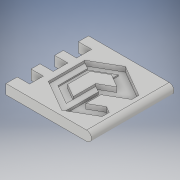
# Autodesk Inventor part: schablone
Saved by Autodesk Inventor 2019 (Build 230136000, 136)
## iProperties
Created: 2019-08-14
Part Number: schablone
Material: Generic
Document SubType Name: Modeling
Designer: Yashar
Density: 1 g/cm^3
Appearance: Default
Author: Yashar
Autodesk Inventor part; units mm, degrees
note: some values were not read from the file. Chosen so that the rebuilt part matches the saved one: direction of "Emboss1".
ref_plane "YZ Plane" through (0, 0, 0) normal (1, 0, 0) x (0, 1, 0)
ref_plane "XZ Plane" through (0, 0, 0) normal (0, 1, 0) x (-1, 0, 0)
ref_plane "XY Plane" through (0, 0, 0) normal (0, 0, 1) x (1, 0, 0)
sketch "Sketch1" plane through (0, 0, 0) normal (0, 1, 0) x (-1, 0, 0)
  line L0 (-17.5, 16.9) -> (17.5, 16.9)
  line L1 (17.5, 16.9) -> (17.5, -16.9)
  line L2 (17.5, -16.9) -> (-17.5, -16.9)
  line L3 (-17.5, -16.9) -> (-17.5, 16.9)
  line L4 (-17.5, 16.9) -> (17.5, -16.9) construction
  line L5 (17.5, 16.9) -> (-17.5, -16.9) construction
  point P0 (0, 0)
  constraints: 12 end point, 2 midpoint, 2 parallel, 1 horizontal, 1 perpendicular
sketch "Sketch2" plane through (0, 0, 0) normal (0, 1, 0) x (-1, 0, 0)
  line L0 (980.2308, 0) -> (977.7308, 0)
  line L1 (17.4632, -0.049) -> (15.105, -0.049)
  line L2 (12.1095, 2.9465) -> (18.1005, 2.9465)
  line L3 (18.1005, 2.9465) -> (18.1005, -3.0446)
  line L4 (18.1005, -3.0446) -> (12.1095, -3.0446)
  line L5 (12.1095, -3.0446) -> (12.1095, 2.9465)
  line L6 (12.1095, 2.9465) -> (18.1005, -3.0446) construction
  line L7 (18.1005, 2.9465) -> (12.1095, -3.0446) construction
  line L8 (12.4632, 12.2678) -> (18.1005, 12.2678)
  line L9 (18.1005, 12.2678) -> (18.1005, 6.638)
  line L10 (18.1005, 6.638) -> (12.4632, 6.638)
  line L11 (12.4632, 6.638) -> (12.4632, 12.2678)
  line L12 (12.4632, 12.2678) -> (18.1005, 6.638) construction
  line L13 (12.0658, -6.5864) -> (18.1005, -6.5864)
  line L14 (18.1005, -6.5864) -> (18.1005, -12.7382)
  line L15 (18.1005, -12.7382) -> (12.0658, -12.7382)
  line L16 (12.0658, -12.7382) -> (12.0658, -6.5864)
  line L17 (12.0658, -6.5864) -> (18.1005, -12.7382) construction
  line L18 (18.1005, -6.5864) -> (12.0658, -12.7382) construction
  point P0 (0, 0)
  dimension "d2" = 2.5
  constraints: 38 end point, 6 parallel, 5 horizontal, 3 perpendicular, 2 midpoint
  measures "d2" distance of L0.start L0.end
extrude "Extrusion1" add sketch "Sketch1" along normal blind 4
extrude "Extrusion2" cut sketch "Sketch2" along normal blind 4
fillet "Fillet3" radius 2 1 edges at (17.5, 4, 0)
fillet "Fillet4" radius 2 1 edges at (17.5, 0, 0)
sketch "Sketch3" plane through (0, 4, 0) normal (0, 1, 0) x (1, 0, 0)
  line L0 (-17.5, 3.0446) -> (-12.1095, 3.0446) construction
  line L1 (-12.1095, 3.0446) -> (-12.1095, -2.9465) construction
  line L2 (-12.1095, -2.9465) -> (-17.5, -2.9465) construction
  line L3 (-17.5, -2.9465) -> (-17.5, -6.638) construction
  line L4 (-17.5, -6.638) -> (-12.4632, -6.638) construction
  line L5 (-12.4632, -6.638) -> (-12.4632, -12.2678) construction
  line L6 (-12.4632, -12.2678) -> (-17.5, -12.2678) construction
  line L7 (-17.5, -12.2678) -> (-17.5, -16.9) construction
  line L8 (-17.5, -16.9) -> (15.5, -16.9) construction
  line L9 (15.5, 16.9) -> (-17.5, 16.9) construction
  line L10 (-17.5, 16.9) -> (-17.5, 12.7382) construction
  line L11 (-17.5, 12.7382) -> (-12.0658, 12.7382) construction
  line L12 (-12.0658, 12.7382) -> (-12.0658, 6.5864) construction
  line L13 (-12.0658, 6.5864) -> (-17.5, 6.5864) construction
  line L14 (-17.5, 6.5864) -> (-17.5, 3.0446) construction
  line L15 (-12.1095, 0.049) -> (15.5, 0) construction
  line L16 (-17.5, 16.9) -> (17.5, 16.9) construction
  line L17 (17.5, -16.9) -> (-17.5, -16.9) construction
  line L18 (-9.5803, 7.5215) -> (-9.5803, -7.4785)
  line L19 (-9.5803, -7.4785) -> (3.41, -14.9785)
  line L20 (-9.5803, 7.5215) -> (-7.0803, 6.0781)
  line L21 (-7.0803, 6.0781) -> (-7.0803, -6.0352)
  line L22 (-7.0803, -6.0352) -> (0.91, -10.6484)
  line L23 (0.91, -10.6484) -> (0.91, 1.4648)
  line L24 (0.91, 1.4648) -> (3.41, 0.0215)
  line L25 (3.41, 0.0215) -> (3.41, -14.9785)
  line L26 (15.5, 16.9) -> (15.5, -16.9) projected
  line L27 (3.41, 16.9) -> (3.41, -16.9) construction
  line L28 (-17.5, -16.9) -> (15.5, -16.9) construction
  line L29 (15.5, 16.9) -> (15.5, 16.9) construction
  line L30 (15.5, 16.9) -> (15.5, -16.9) construction
  line L31 (15.5, -16.9) -> (15.5, -16.9) construction
  line L32 (15.5, -16.9) -> (15.5, 16.9) construction
  dimension "d23" = 2.5
  dimension "d24" = 2.5
  dimension "d25" = 2.5
  dimension "d26" = 15
  dimension "d28" = 15
  constraints: 20 end point, 4 parallel, 3 collinear, 3 point on line, 2 midpoint, 1 perpendicular, 1 vertical
  measures "d23" distance between parallel lines of L21 L18
  measures "d24" distance between parallel lines of L25 L23
  measures "d25" distance between parallel lines of L19 L22
  measures "d26" distance of L18.start L18.end
  measures "d28" distance of L18.end L19.end
emboss "Emboss1" sketch "Sketch3" operation cut depth 1 direction (0, -1, 0)
sketch "Sketch4" plane through (0, 4, 0) normal (0, 1, 0) x (1, 0, 0)
  line L0 (-9.5803, 7.5215) -> (-7.0803, 6.0781) construction
  line L1 (-7.0803, 6.0781) -> (-7.0803, -6.0352) construction
  line L2 (-7.0803, -6.0352) -> (0.91, -10.6484) construction
  line L3 (0.91, -10.6484) -> (0.91, 1.4648) construction
  line L4 (0.91, 1.4648) -> (3.41, 0.0215) construction
  line L5 (3.41, 0.0215) -> (3.41, -14.9785) construction
  line L6 (3.41, -14.9785) -> (-9.5803, -7.4785) construction
  line L7 (-9.5803, -7.4785) -> (-9.5803, 7.5215) construction
  line L8 (15.5, 16.9) -> (15.5, -16.9) construction
  line L9 (15.5, 16.9) -> (-17.5, 16.9) construction
  line L10 (-17.5, 16.9) -> (-17.5, 12.7382) construction
  line L11 (-17.5, 12.7382) -> (-12.0658, 12.7382) construction
  line L12 (-12.0658, 12.7382) -> (-12.0658, 6.5864) construction
  line L13 (-12.0658, 6.5864) -> (-17.5, 6.5864) construction
  line L14 (-17.5, 6.5864) -> (-17.5, 3.0446) construction
  line L15 (-17.5, 3.0446) -> (-12.1095, 3.0446) construction
  line L16 (-12.1095, 3.0446) -> (-12.1095, -2.9465) construction
  line L17 (-12.1095, -2.9465) -> (-17.5, -2.9465) construction
  line L18 (-17.5, -2.9465) -> (-17.5, -6.638) construction
  line L19 (-17.5, -6.638) -> (-12.4632, -6.638) construction
  line L20 (-12.4632, -6.638) -> (-12.4632, -12.2678) construction
  line L21 (-12.4632, -12.2678) -> (-17.5, -12.2678) construction
  line L22 (-17.5, -12.2678) -> (-17.5, -16.9) construction
  line L23 (-17.5, -16.9) -> (15.5, -16.9) construction
  line L24 (-12.1095, 0.049) -> (15.5, 0) construction
  line L25 (15.5, -16.9) -> (15.5, 16.9) construction
  line L26 (0.91, 16.9) -> (0.91, -16.9) construction
  line L27 (15.5, -16.9) -> (-17.5, -16.9) construction
  line L28 (0.91, -10.6484) -> (0.91, 1.4648) construction
  line L29 (-7.0803, 6.0781) -> (-7.0803, -6.0352) projected
  line L30 (-7.0803, -6.0352) -> (0.91, -10.6484) projected
  line L31 (-7.0803, 6.0781) -> (-7.0803, -6.0352)
  line L32 (-7.0803, -6.0352) -> (0.91, -10.6484)
  line L33 (0.91, -10.6484) -> (0.91, -7.7617)
  line L34 (0.91, -10.6484) -> (0.91, 1.4648) projected
  line L35 (0.91, -7.7617) -> (-4.5803, -4.5918)
  line L36 (-4.5803, -4.5918) -> (-4.5803, 4.6347)
  line L37 (-4.5803, 4.6347) -> (0.91, 7.8046)
  line L38 (-7.0803, 6.0781) -> (0.91, 10.6913)
  line L39 (0.91, 10.6913) -> (0.91, 7.8046)
  point P0 (0, 0)
  dimension "d29" = 120
  dimension "d30" = 2.5
  dimension "d31" = 2.5
  dimension "d32" = 2.5
  constraints: 20 end point, 5 point on line, 4 collinear, 4 parallel, 2 midpoint
  measures "d29" angle of L38 L0
  measures "d30" distance between parallel lines of L1 L36
  measures "d31" distance between parallel lines of L38 L37
  measures "d32" distance between parallel lines of L2 L35
emboss "Emboss2" sketch "Sketch4" operation cut depth 1.5 direction (0, -1, 0)
sketch "Sketch5" plane through (0, 4, 0) normal (0, 1, 0) x (1, 0, 0)
  line L0 (-4.5803, -4.5918) -> (0.91, -7.7617) construction
  line L1 (0.91, -7.7617) -> (0.91, 1.4648) construction
  line L2 (0.91, 1.4648) -> (3.41, 0.0215) construction
  line L3 (3.41, 0.0215) -> (3.41, -14.9785) construction
  line L4 (3.41, -14.9785) -> (-9.5803, -7.4785) construction
  line L5 (-9.5803, -7.4785) -> (-9.5803, 7.5215) construction
  line L6 (-9.5803, 7.5215) -> (-7.0803, 6.0781) construction
  line L7 (-7.0803, 6.0781) -> (0.91, 10.6913) construction
  line L8 (0.91, 10.6913) -> (0.91, 7.8046) construction
  line L9 (0.91, 7.8046) -> (-4.5803, 4.6347) construction
  line L10 (-4.5803, 4.6347) -> (-4.5803, -4.5918) construction
  line L11 (15.5, 16.9) -> (15.5, -16.9) construction
  line L12 (15.5, 16.9) -> (-17.5, 16.9) construction
  line L13 (-17.5, 16.9) -> (-17.5, 12.7382) construction
  line L14 (-17.5, 12.7382) -> (-12.0658, 12.7382) construction
  line L15 (-12.0658, 12.7382) -> (-12.0658, 6.5864) construction
  line L16 (-12.0658, 6.5864) -> (-17.5, 6.5864) construction
  line L17 (-17.5, 6.5864) -> (-17.5, 3.0446) construction
  line L18 (-17.5, 3.0446) -> (-12.1095, 3.0446) construction
  line L19 (-12.1095, 3.0446) -> (-12.1095, -2.9465) construction
  line L20 (-12.1095, -2.9465) -> (-17.5, -2.9465) construction
  line L21 (-17.5, -2.9465) -> (-17.5, -6.638) construction
  line L22 (-17.5, -6.638) -> (-12.4632, -6.638) construction
  line L23 (-12.4632, -6.638) -> (-12.4632, -12.2678) construction
  line L24 (-12.4632, -12.2678) -> (-17.5, -12.2678) construction
  line L25 (-17.5, -12.2678) -> (-17.5, -16.9) construction
  line L26 (-17.5, -16.9) -> (15.5, -16.9) construction
  line L27 (-7.0803, 6.0781) -> (0.91, 10.6913) projected
  line L28 (-9.5803, 7.5215) -> (-7.0803, 6.0781)
  line L29 (-7.0803, 6.0781) -> (0.91, 10.6913)
  line L30 (0.91, 10.6913) -> (0.91, 7.8046)
  line L31 (0.91, 10.6913) -> (0.91, 7.8046) projected
  line L32 (0.91, 16.9) -> (0.91, -16.9) construction
  line L33 (0.91, -7.7617) -> (0.91, 1.4648) construction
  line L34 (-9.5803, 7.5215) -> (0.91, 13.5781)
  line L35 (0.91, 13.5781) -> (13.9004, 6.0781)
  line L36 (13.9004, 6.0781) -> (13.9004, 3.1913)
  line L37 (13.9004, 3.1913) -> (5.91, -1.4219)
  line L38 (5.91, -1.4219) -> (5.91, -7.6363)
  line L39 (5.91, -7.6363) -> (11.2919, -4.5291)
  line L40 (13.9004, -6.0352) -> (13.9004, -8.9219)
  line L41 (3.41, -14.9785) -> (-9.5803, -7.4785) projected
  line L42 (13.9004, -8.9219) -> (3.41, -14.9785)
  line L43 (0.91, 1.4648) -> (3.41, 0.0215) projected
  line L44 (3.41, -14.9785) -> (3.41, 0.0215)
  line L45 (3.41, 0.0215) -> (0.91, 1.4648)
  line L46 (0.91, 7.8046) -> (-4.5803, 4.6347) projected
  line L47 (0.91, 7.8046) -> (0.91, 10.6913)
  line L48 (3.41, 0.0215) -> (3.41, -14.9785) projected
  line L49 (0.91, 1.4648) -> (6.4004, 4.6347)
  line L50 (6.4004, 4.6347) -> (0.91, 7.8046)
  line L51 (13.9004, -6.0352) -> (11.2919, -4.5291)
  line L52 (-7.1521, -6.1594) -> (3.41, -12.0918) construction
  line L53 (-4.5803, -4.5918) -> (0.91, -7.7617) construction
  line L54 (-4.5803, -4.5918) -> (3.41, -9.0797) construction
  line L55 (3.41, -9.0797) -> (14.5341, -2.6572) construction
  line L56 (3.41, 0.0215) -> (13.9004, 6.0781) construction
  line L57 (3.41, -12.0918) -> (19.1495, -3.0046) construction
  line L58 (6.4004, 4.6347) -> (9.227, 5.8895) construction
  line L59 (0.91, 10.6913) -> (0.91, 7.8046) construction
  line L60 (9.227, 5.8895) -> (0.91, 10.6913) construction
  point P0 (0, 0)
  dimension "d35" = 60
  dimension "d36" = 2.5
  dimension "d39" = 120
  dimension "d42" = 120
  dimension "d43" = 2.5
  constraints: 50 end point, 12 parallel, 7 point on line, 5 collinear, 1 vertical, 1 other
  measures "d35" angle of L6 L34
  measures "d36" distance between parallel lines of L38 L3
  measures "d39" angle of L32 L35
  measures "d42" angle of L3 L55
  measures "d43" distance between parallel lines of L56 L37
emboss "Emboss3" sketch "Sketch5" operation cut depth 2 direction (0, -1, 0)
equation "\"d24\" = d23"
equation "\"d25\" = d23"
equation "\"d28\" = d26"
equation "\"d30\" = d23"
equation "\"d31\" = d23"
equation "\"d32\" = d23"
equation "\"d36\" = d23"
equation "\"d43\" = d23"
body "Solid1"
